Autodesk Fusion 360 part; units mm, degrees
(part 2 of 7)
sketch "Cover bearing-pad clearance sketch (3)" plane through (0, 0, 39.1) normal (0, 0, 1) x (1, 0, 0) in component "01 Shape A housing"
  circle A0 centre (77, 172) radius 4.9
  dimension "d450" = 77
  dimension "d451" = 172
  dimension "d452" = 4.9
  measures "d450" horizontal distance of origin A0.centre
  measures "d451" vertical distance of origin A0.centre
  measures "d452" radius of A0
ref_plane "WorkPlane1" through (0, 0, -8) normal (0, 0, 1) x (1, 0, 0) in component "M3 x 8 button screw — GEN-M3-BHCS-L8-AF2"
sketch "Joined screw sketch" plane through (0, 0, -8) normal (0, 0, 1) x (1, 0, 0) in component "M3 x 8 button screw — GEN-M3-BHCS-L8-AF2"
  circle A0 centre (0, 0) radius 1.45
  dimension "d457" = 1.45
  measures "d457" radius of A0
extrude "Joined screw" add sketch "Joined screw sketch" along normal blind 8 separate body makes body 17 in component "M3 x 8 button screw — GEN-M3-BHCS-L8-AF2"
ref_plane "WorkPlane2" through (0, 0, 0) normal (0, 0, 1) x (1, 0, 0) in component "M3 x 8 button screw — GEN-M3-BHCS-L8-AF2"
sketch "Screw head sketch" plane through (0, 0, 0) normal (0, 0, 1) x (1, 0, 0) in component "M3 x 8 button screw — GEN-M3-BHCS-L8-AF2"
  circle A0 centre (0, 0) radius 2.85
  dimension "d462" = 2.85
  measures "d462" radius of A0
extrude "Screw head" add sketch "Screw head sketch" along normal blind 1.65 bodies 17 in component "M3 x 8 button screw — GEN-M3-BHCS-L8-AF2"
fillet "Rounded head crown" radius 0.95 1 edges at (-2.6571, -1.0306, 1.65) on bodies 17 in component "M3 x 8 button screw — GEN-M3-BHCS-L8-AF2"
ref_plane "WorkPlane3" through (0, 0, 0.65) normal (0, 0, 1) x (1, 0, 0) in component "M3 x 8 button screw — GEN-M3-BHCS-L8-AF2"
sketch "Hex drive 2 mm across flats" plane through (0, 0, 0.65) normal (0, 0, 1) x (1, 0, 0) in component "M3 x 8 button screw — GEN-M3-BHCS-L8-AF2"
  line L0 (1.1547, 0) -> (0.5774, 1)
  line L1 (0.5774, 1) -> (-0.5774, 1)
  line L2 (-0.5774, 1) -> (-1.1547, 0)
  line L3 (-1.1547, 0) -> (-0.5774, -1)
  line L4 (-0.5774, -1) -> (0.5774, -1)
  line L5 (0.5774, -1) -> (1.1547, 0)
extrude "Hex drive recess" cut sketch "Hex drive 2 mm across flats" along normal blind 1.1 bodies 17 in component "M3 x 8 button screw — GEN-M3-BHCS-L8-AF2"
ref_plane "WorkPlane1" through (0, 0, -5) normal (0, 0, 1) x (1, 0, 0) in component "M3 insert OD4.2 x5 — GEN-M3-HEATSET-OD4.2-L5"
sketch "Hollow insert sketch" plane through (0, 0, -5) normal (0, 0, 1) x (1, 0, 0) in component "M3 insert OD4.2 x5 — GEN-M3-HEATSET-OD4.2-L5"
  circle A0 centre (0, 0) radius 2.1
  dimension "d473" = 2.1
  measures "d473" radius of A0
extrude "Hollow insert" add sketch "Hollow insert sketch" along normal blind 5 separate body makes body 18 in component "M3 insert OD4.2 x5 — GEN-M3-HEATSET-OD4.2-L5"
ref_plane "WorkPlane2" through (0, 0, -5.1) normal (0, 0, 1) x (1, 0, 0) in component "M3 insert OD4.2 x5 — GEN-M3-HEATSET-OD4.2-L5"
sketch "Unthreaded insert bore sketch" plane through (0, 0, -5.1) normal (0, 0, 1) x (1, 0, 0) in component "M3 insert OD4.2 x5 — GEN-M3-HEATSET-OD4.2-L5"
  circle A0 centre (0, 0) radius 1.55
  dimension "d478" = 1.55
  measures "d478" radius of A0
extrude "Unthreaded insert bore" cut sketch "Unthreaded insert bore sketch" along normal blind 5.2 bodies 18 in component "M3 insert OD4.2 x5 — GEN-M3-HEATSET-OD4.2-L5"
ref_plane "WorkPlane3" through (0, 0, -3.75) normal (0, 0, 1) x (1, 0, 0) in component "M3 insert OD4.2 x5 — GEN-M3-HEATSET-OD4.2-L5"
sketch "Cosmetic insert relief" plane through (0, 0, -3.75) normal (0, 0, 1) x (1, 0, 0) in component "M3 insert OD4.2 x5 — GEN-M3-HEATSET-OD4.2-L5"
  circle A0 centre (0, 0) radius 2.2
  circle A1 centre (0, 0) radius 2
  dimension "d483" = 2.2
  dimension "d484" = 2
  measures "d483" radius of A0
  measures "d484" radius of A1
extrude "Cosmetic annular relief" cut sketch "Cosmetic insert relief" along normal blind 0.25 bodies 18 in component "M3 insert OD4.2 x5 — GEN-M3-HEATSET-OD4.2-L5"
ref_plane "WorkPlane4" through (0, 0, -1.25) normal (0, 0, 1) x (1, 0, 0) in component "M3 insert OD4.2 x5 — GEN-M3-HEATSET-OD4.2-L5"
sketch "Cosmetic insert relief (1)" plane through (0, 0, -1.25) normal (0, 0, 1) x (1, 0, 0) in component "M3 insert OD4.2 x5 — GEN-M3-HEATSET-OD4.2-L5"
  circle A0 centre (0, 0) radius 2.2
  circle A1 centre (0, 0) radius 2
  dimension "d489" = 2.2
  dimension "d490" = 2
  measures "d489" radius of A0
  measures "d490" radius of A1
extrude "Cosmetic annular relief (1)" cut sketch "Cosmetic insert relief (1)" along normal blind 0.25 bodies 18 in component "M3 insert OD4.2 x5 — GEN-M3-HEATSET-OD4.2-L5"
ref_plane "WorkPlane14" through (0, 0, 38.6) normal (0, 0, 1) x (1, 0, 0) in component "02 Single rear cover"
sketch "Rear cover locating lip sketch" plane through (0, 0, 38.6) normal (0, 0, 1) x (1, 0, 0) in component "02 Single rear cover"
  line L0 (2.65, 55) -> (4.65, 55)
  line L1 (4.65, 55) -> (4.65, 67)
  line L2 (4.65, 67) -> (2.65, 67)
  line L3 (2.65, 67) -> (2.65, 55)
  dimension "d495" = 2.65
  dimension "d496" = 55
  dimension "d497" = 2
  dimension "d498" = 12
  constraint horizontal L0
  constraint vertical L1
  constraint horizontal L2
  constraint vertical L3
  measures "d495" horizontal distance of origin L0.start
  measures "d496" vertical distance of origin L0.start
  measures "d497" horizontal distance of L0.start L0.end
  measures "d498" vertical distance of L0.end L1.end
extrude "Rear cover locating lip" add sketch "Rear cover locating lip sketch" along normal blind 2.3 bodies 4 in component "02 Single rear cover"
ref_plane "WorkPlane15" through (0, 0, 38.6) normal (0, 0, 1) x (1, 0, 0) in component "02 Single rear cover"
sketch "Rear cover locating lip sketch (1)" plane through (0, 0, 38.6) normal (0, 0, 1) x (1, 0, 0) in component "02 Single rear cover"
  line L0 (2.65, 98) -> (4.65, 98)
  line L1 (4.65, 98) -> (4.65, 110)
  line L2 (4.65, 110) -> (2.65, 110)
  line L3 (2.65, 110) -> (2.65, 98)
  dimension "d503" = 2.65
  dimension "d504" = 98
  dimension "d505" = 2
  dimension "d506" = 12
  constraint horizontal L0
  constraint vertical L1
  constraint horizontal L2
  constraint vertical L3
  measures "d503" horizontal distance of origin L0.start
  measures "d504" vertical distance of origin L0.start
  measures "d505" horizontal distance of L0.start L0.end
  measures "d506" vertical distance of L0.end L1.end
extrude "Rear cover locating lip (1)" add sketch "Rear cover locating lip sketch (1)" along normal blind 2.3 bodies 4 in component "02 Single rear cover"
ref_plane "WorkPlane16" through (0, 0, 38.6) normal (0, 0, 1) x (1, 0, 0) in component "02 Single rear cover"
sketch "Rear cover locating lip sketch (2)" plane through (0, 0, 38.6) normal (0, 0, 1) x (1, 0, 0) in component "02 Single rear cover"
  line L0 (80.35, 55) -> (82.35, 55)
  line L1 (82.35, 55) -> (82.35, 67)
  line L2 (82.35, 67) -> (80.35, 67)
  line L3 (80.35, 67) -> (80.35, 55)
  dimension "d511" = 80.35
  dimension "d512" = 55
  dimension "d513" = 2
  dimension "d514" = 12
  constraint horizontal L0
  constraint vertical L1
  constraint horizontal L2
  constraint vertical L3
  measures "d511" horizontal distance of origin L0.start
  measures "d512" vertical distance of origin L0.start
  measures "d513" horizontal distance of L0.start L0.end
  measures "d514" vertical distance of L0.end L1.end
extrude "Rear cover locating lip (2)" add sketch "Rear cover locating lip sketch (2)" along normal blind 2.3 bodies 4 in component "02 Single rear cover"
ref_plane "WorkPlane17" through (0, 0, 38.6) normal (0, 0, 1) x (1, 0, 0) in component "02 Single rear cover"
sketch "Rear cover locating lip sketch (3)" plane through (0, 0, 38.6) normal (0, 0, 1) x (1, 0, 0) in component "02 Single rear cover"
  line L0 (80.35, 98) -> (82.35, 98)
  line L1 (82.35, 98) -> (82.35, 110)
  line L2 (82.35, 110) -> (80.35, 110)
  line L3 (80.35, 110) -> (80.35, 98)
  dimension "d519" = 80.35
  dimension "d520" = 98
  dimension "d521" = 2
  dimension "d522" = 12
  constraint horizontal L0
  constraint vertical L1
  constraint horizontal L2
  constraint vertical L3
  measures "d519" horizontal distance of origin L0.start
  measures "d520" vertical distance of origin L0.start
  measures "d521" horizontal distance of L0.start L0.end
  measures "d522" vertical distance of L0.end L1.end
extrude "Rear cover locating lip (3)" add sketch "Rear cover locating lip sketch (3)" along normal blind 2.3 bodies 4 in component "02 Single rear cover"
ref_plane "WorkPlane24" through (0, 0, 14.3) normal (0, 0, 1) x (1, 0, 0) in component "01 Shape A housing"
sketch "Lower battery cradle and divider anchor sketch" plane through (0, 0, 14.3) normal (0, 0, 1) x (1, 0, 0) in component "01 Shape A housing"
  line L0 (2.3, 24.5) -> (50.2, 24.5)
  line L1 (50.2, 24.5) -> (50.2, 26.5)
  line L2 (50.2, 26.5) -> (2.3, 26.5)
  line L3 (2.3, 26.5) -> (2.3, 24.5)
  dimension "d527" = 2.3
  dimension "d528" = 24.5
  dimension "d529" = 47.9
  dimension "d530" = 2
  constraint horizontal L0
  constraint vertical L1
  constraint horizontal L2
  constraint vertical L3
  measures "d527" horizontal distance of origin L0.start
  measures "d528" vertical distance of origin L0.start
  measures "d529" horizontal distance of L0.start L0.end
  measures "d530" vertical distance of L0.end L1.end
extrude "Lower battery cradle and divider anchor" add sketch "Lower battery cradle and divider anchor sketch" along normal blind 4.2 bodies 1 in component "01 Shape A housing"
ref_plane "WorkPlane25" through (0, 0, 14.3) normal (0, 0, 1) x (1, 0, 0) in component "01 Shape A housing"
sketch "Battery to PCB guide divider sketch" plane through (0, 0, 14.3) normal (0, 0, 1) x (1, 0, 0) in component "01 Shape A housing"
  line L0 (48.2, 25) -> (50.2, 25)
  line L1 (50.2, 25) -> (50.2, 117.6)
  line L2 (50.2, 117.6) -> (48.2, 117.6)
  line L3 (48.2, 117.6) -> (48.2, 25)
  dimension "d535" = 48.2
  dimension "d536" = 25
  dimension "d537" = 2
  dimension "d538" = 92.6
  constraint horizontal L0
  constraint vertical L1
  constraint horizontal L2
  constraint vertical L3
  measures "d535" horizontal distance of origin L0.start
  measures "d536" vertical distance of origin L0.start
  measures "d537" horizontal distance of L0.start L0.end
  measures "d538" vertical distance of L0.end L1.end
extrude "Battery to PCB guide divider" add sketch "Battery to PCB guide divider sketch" along normal blind 21.7 bodies 1 in component "01 Shape A housing"
ref_plane "WorkPlane26" through (0, 0, 14.3) normal (0, 0, 1) x (1, 0, 0) in component "01 Shape A housing"
sketch "Carrier fixed support web sketch" plane through (0, 0, 14.3) normal (0, 0, 1) x (1, 0, 0) in component "01 Shape A housing"
  line L0 (72.4, 24.4) -> (82.7, 24.4)
  line L1 (82.7, 24.4) -> (82.7, 31.6)
  line L2 (82.7, 31.6) -> (72.4, 31.6)
  line L3 (72.4, 31.6) -> (72.4, 24.4)
  dimension "d543" = 72.4
  dimension "d544" = 24.4
  dimension "d545" = 10.3
  dimension "d546" = 7.2
  constraint horizontal L0
  constraint vertical L1
  constraint horizontal L2
  constraint vertical L3
  measures "d543" horizontal distance of origin L0.start
  measures "d544" vertical distance of origin L0.start
  measures "d545" horizontal distance of L0.start L0.end
  measures "d546" vertical distance of L0.end L1.end
extrude "Carrier fixed support web" add sketch "Carrier fixed support web sketch" along normal blind 4.2 bodies 1 in component "01 Shape A housing"
ref_plane "WorkPlane27" through (0, 0, 14.4) normal (0, 0, 1) x (1, 0, 0) in component "01 Shape A housing"
sketch "Carrier M2 insert pilot sketch" plane through (0, 0, 14.4) normal (0, 0, 1) x (1, 0, 0) in component "01 Shape A housing"
  circle A0 centre (76, 28) radius 1.65
  dimension "d551" = 76
  dimension "d552" = 28
  dimension "d553" = 1.65
  measures "d551" horizontal distance of origin A0.centre
  measures "d552" vertical distance of origin A0.centre
  measures "d553" radius of A0
extrude "Carrier M2 insert pilot" cut sketch "Carrier M2 insert pilot sketch" along normal blind 4.2 bodies 1 in component "01 Shape A housing"
ref_plane "WorkPlane28" through (0, 0, 14.3) normal (0, 0, 1) x (1, 0, 0) in component "01 Shape A housing"
sketch "Carrier fixed support web sketch (1)" plane through (0, 0, 14.3) normal (0, 0, 1) x (1, 0, 0) in component "01 Shape A housing"
  line L0 (48.2, 110.4) -> (58.4, 110.4)
  line L1 (58.4, 110.4) -> (58.4, 117.6)
  line L2 (58.4, 117.6) -> (48.2, 117.6)
  line L3 (48.2, 117.6) -> (48.2, 110.4)
  dimension "d558" = 48.2
  dimension "d559" = 110.4
  dimension "d560" = 10.2
  dimension "d561" = 7.2
  constraint horizontal L0
  constraint vertical L1
  constraint horizontal L2
  constraint vertical L3
  measures "d558" horizontal distance of origin L0.start
  measures "d559" vertical distance of origin L0.start
  measures "d560" horizontal distance of L0.start L0.end
  measures "d561" vertical distance of L0.end L1.end
extrude "Carrier fixed support web (1)" add sketch "Carrier fixed support web sketch (1)" along normal blind 4.2 bodies 1 in component "01 Shape A housing"
ref_plane "WorkPlane29" through (0, 0, 14.4) normal (0, 0, 1) x (1, 0, 0) in component "01 Shape A housing"
sketch "Carrier M2 insert pilot sketch (1)" plane through (0, 0, 14.4) normal (0, 0, 1) x (1, 0, 0) in component "01 Shape A housing"
  circle A0 centre (54.8, 114) radius 1.65
  dimension "d566" = 54.8
  dimension "d567" = 114
  dimension "d568" = 1.65
  measures "d566" horizontal distance of origin A0.centre
  measures "d567" vertical distance of origin A0.centre
  measures "d568" radius of A0
extrude "Carrier M2 insert pilot (1)" cut sketch "Carrier M2 insert pilot sketch (1)" along normal blind 4.2 bodies 1 in component "01 Shape A housing"
ref_plane "WorkPlane1" through (0, 0, 18.5) normal (0, 0, 1) x (1, 0, 0) in component "Carrier / removable electronics tray"
sketch "PCB carrier plate sketch" plane through (0, 0, 18.5) normal (0, 0, 1) x (1, 0, 0) in component "Carrier / removable electronics tray"
  line L0 (50.2, 20.5) -> (80.6, 20.5)
  line L1 (80.6, 20.5) -> (80.6, 120.5)
  line L2 (80.6, 120.5) -> (50.2, 120.5)
  line L3 (50.2, 120.5) -> (50.2, 20.5)
  dimension "d573" = 50.2
  dimension "d574" = 20.5
  dimension "d575" = 30.4
  dimension "d576" = 100
  constraint horizontal L0
  constraint vertical L1
  constraint horizontal L2
  constraint vertical L3
  measures "d573" horizontal distance of origin L0.start
  measures "d574" vertical distance of origin L0.start
  measures "d575" horizontal distance of L0.start L0.end
  measures "d576" vertical distance of L0.end L1.end
extrude "PCB carrier plate" add sketch "PCB carrier plate sketch" along normal blind 2 separate body makes body 19 in component "Carrier / removable electronics tray"
ref_plane "WorkPlane1" through (0, 0, 20.5) normal (0, 0, 1) x (1, 0, 0) in component "Carrier / future PCB allocation — layout pending"
sketch "Future shaped PCB sketch" plane through (0, 0, 20.5) normal (0, 0, 1) x (1, 0, 0) in component "Carrier / future PCB allocation — layout pending"
  line L0 (50.4, 21) -> (80.4, 21)
  line L1 (80.4, 21) -> (80.4, 120)
  line L2 (80.4, 120) -> (50.4, 120)
  line L3 (50.4, 120) -> (50.4, 21)
  dimension "d581" = 50.4
  dimension "d582" = 21
  dimension "d583" = 30
  dimension "d584" = 99
  constraint horizontal L0
  constraint vertical L1
  constraint horizontal L2
  constraint vertical L3
  measures "d581" horizontal distance of origin L0.start
  measures "d582" vertical distance of origin L0.start
  measures "d583" horizontal distance of L0.start L0.end
  measures "d584" vertical distance of L0.end L1.end
extrude "Future shaped PCB" add sketch "Future shaped PCB sketch" along normal blind 1.6 separate body makes body 20 in component "Carrier / future PCB allocation — layout pending"
ref_plane "WorkPlane2" through (0, 0, 18.4) normal (0, 0, 1) x (1, 0, 0) in component "Carrier / removable electronics tray"
sketch "Button terminal and finger access notch sketch" plane through (0, 0, 18.4) normal (0, 0, 1) x (1, 0, 0) in component "Carrier / removable electronics tray"
  line L0 (59, 103) -> (89, 103)
  line L1 (89, 103) -> (89, 121)
  line L2 (89, 121) -> (59, 121)
  line L3 (59, 121) -> (59, 103)
  dimension "d589" = 59
  dimension "d590" = 103
  dimension "d591" = 30
  dimension "d592" = 18
  constraint horizontal L0
  constraint vertical L1
  constraint horizontal L2
  constraint vertical L3
  measures "d589" horizontal distance of origin L0.start
  measures "d590" vertical distance of origin L0.start
  measures "d591" horizontal distance of L0.start L0.end
  measures "d592" vertical distance of L0.end L1.end
extrude "Button terminal and finger access notch" cut sketch "Button terminal and finger access notch sketch" along normal blind 4 bodies 19 in component "Carrier / removable electronics tray"
ref_plane "WorkPlane3" through (0, 0, 18.4) normal (0, 0, 1) x (1, 0, 0) in component "Carrier / removable electronics tray"
sketch "Shared carrier M2 hole sketch" plane through (0, 0, 18.4) normal (0, 0, 1) x (1, 0, 0) in component "Carrier / removable electronics tray"
  circle A0 centre (76, 28) radius 1.15
  dimension "d597" = 76
  dimension "d598" = 28
  dimension "d599" = 1.15
  measures "d597" horizontal distance of origin A0.centre
  measures "d598" vertical distance of origin A0.centre
  measures "d599" radius of A0
extrude "Shared carrier M2 hole" cut sketch "Shared carrier M2 hole sketch" along normal blind 4 bodies 19 in component "Carrier / removable electronics tray"
ref_plane "WorkPlane4" through (0, 0, 18.4) normal (0, 0, 1) x (1, 0, 0) in component "Carrier / removable electronics tray"
sketch "Shared carrier M2 hole sketch (1)" plane through (0, 0, 18.4) normal (0, 0, 1) x (1, 0, 0) in component "Carrier / removable electronics tray"
  circle A0 centre (54.8, 114) radius 1.15
  dimension "d604" = 54.8
  dimension "d605" = 114
  dimension "d606" = 1.15
  measures "d604" horizontal distance of origin A0.centre
  measures "d605" vertical distance of origin A0.centre
  measures "d606" radius of A0
extrude "Shared carrier M2 hole (1)" cut sketch "Shared carrier M2 hole sketch (1)" along normal blind 4 bodies 19 in component "Carrier / removable electronics tray"
ref_plane "WorkPlane2" through (0, 0, 18.4) normal (0, 0, 1) x (1, 0, 0) in component "Carrier / future PCB allocation — layout pending"
sketch "Button terminal and finger access notch sketch (2)" plane through (0, 0, 18.4) normal (0, 0, 1) x (1, 0, 0) in component "Carrier / future PCB allocation — layout pending"
  line L0 (59, 103) -> (89, 103)
  line L1 (89, 103) -> (89, 121)
  line L2 (89, 121) -> (59, 121)
  line L3 (59, 121) -> (59, 103)
  dimension "d611" = 59
  dimension "d612" = 103
  dimension "d613" = 30
  dimension "d614" = 18
  constraint horizontal L0
  constraint vertical L1
  constraint horizontal L2
  constraint vertical L3
  measures "d611" horizontal distance of origin L0.start
  measures "d612" vertical distance of origin L0.start
  measures "d613" horizontal distance of L0.start L0.end
  measures "d614" vertical distance of L0.end L1.end
extrude "Button terminal and finger access notch'" cut sketch "Button terminal and finger access notch sketch (2)" along normal blind 4 bodies 20 in component "Carrier / future PCB allocation — layout pending"
ref_plane "WorkPlane3" through (0, 0, 18.4) normal (0, 0, 1) x (1, 0, 0) in component "Carrier / future PCB allocation — layout pending"
sketch "Shared carrier M2 hole sketch (2)" plane through (0, 0, 18.4) normal (0, 0, 1) x (1, 0, 0) in component "Carrier / future PCB allocation — layout pending"
  circle A0 centre (76, 28) radius 1.15
  dimension "d619" = 76
  dimension "d620" = 28
  dimension "d621" = 1.15
  measures "d619" horizontal distance of origin A0.centre
  measures "d620" vertical distance of origin A0.centre
  measures "d621" radius of A0
extrude "Shared carrier M2 hole'" cut sketch "Shared carrier M2 hole sketch (2)" along normal blind 4 bodies 20 in component "Carrier / future PCB allocation — layout pending"
ref_plane "WorkPlane4" through (0, 0, 18.4) normal (0, 0, 1) x (1, 0, 0) in component "Carrier / future PCB allocation — layout pending"
sketch "Shared carrier M2 hole sketch (1) (2)" plane through (0, 0, 18.4) normal (0, 0, 1) x (1, 0, 0) in component "Carrier / future PCB allocation — layout pending"
  circle A0 centre (54.8, 114) radius 1.15
  dimension "d626" = 54.8
  dimension "d627" = 114
  dimension "d628" = 1.15
  measures "d626" horizontal distance of origin A0.centre
  measures "d627" vertical distance of origin A0.centre
  measures "d628" radius of A0
extrude "Shared carrier M2 hole (1)'" cut sketch "Shared carrier M2 hole sketch (1) (2)" along normal blind 4 bodies 20 in component "Carrier / future PCB allocation — layout pending"
ref_plane "WorkPlane5" through (0, 0, 22.1) normal (0, 0, 1) x (1, 0, 0) in component "Carrier / future PCB allocation — layout pending"
sketch "Charger power zone sketch" plane through (0, 0, 22.1) normal (0, 0, 1) x (1, 0, 0) in component "Carrier / future PCB allocation — layout pending"
  line L0 (54, 37) -> (74, 37)
  line L1 (74, 37) -> (74, 60)
  line L2 (74, 60) -> (54, 60)
  line L3 (54, 60) -> (54, 37)
  dimension "d633" = 54
  dimension "d634" = 37
  dimension "d635" = 20
  dimension "d636" = 23
  constraint horizontal L0
  constraint vertical L1
  constraint horizontal L2
  constraint vertical L3
  measures "d633" horizontal distance of origin L0.start
  measures "d634" vertical distance of origin L0.start
  measures "d635" horizontal distance of L0.start L0.end
  measures "d636" vertical distance of L0.end L1.end
extrude "Charger power zone" add sketch "Charger power zone sketch" along normal blind 5 separate body makes body 21 in component "Carrier / future PCB allocation — layout pending"
ref_plane "WorkPlane6" through (0, 0, 22.1) normal (0, 0, 1) x (1, 0, 0) in component "Carrier / future PCB allocation — layout pending"
sketch "Sensor analog zone sketch" plane through (0, 0, 22.1) normal (0, 0, 1) x (1, 0, 0) in component "Carrier / future PCB allocation — layout pending"
  line L0 (54, 68) -> (74, 68)
  line L1 (74, 68) -> (74, 88)
  line L2 (74, 88) -> (54, 88)
  line L3 (54, 88) -> (54, 68)
  dimension "d641" = 54
  dimension "d642" = 68
  dimension "d643" = 20
  dimension "d644" = 20
  constraint horizontal L0
  constraint vertical L1
  constraint horizontal L2
  constraint vertical L3
  measures "d641" horizontal distance of origin L0.start
  measures "d642" vertical distance of origin L0.start
  measures "d643" horizontal distance of L0.start L0.end
  measures "d644" vertical distance of L0.end L1.end
extrude "Sensor analog zone" add sketch "Sensor analog zone sketch" along normal blind 4 separate body makes body 22 in component "Carrier / future PCB allocation — layout pending"
ref_plane "WorkPlane7" through (0, 0, 22.1) normal (0, 0, 1) x (1, 0, 0) in component "Carrier / future PCB allocation — layout pending"
sketch "Digital interface zone sketch" plane through (0, 0, 22.1) normal (0, 0, 1) x (1, 0, 0) in component "Carrier / future PCB allocation — layout pending"
  line L0 (54, 94) -> (72, 94)
  line L1 (72, 94) -> (72, 102)
  line L2 (72, 102) -> (54, 102)
  line L3 (54, 102) -> (54, 94)
  dimension "d649" = 54
  dimension "d650" = 94
  dimension "d651" = 18
  dimension "d652" = 8
  constraint horizontal L0
  constraint vertical L1
  constraint horizontal L2
  constraint vertical L3
  measures "d649" horizontal distance of origin L0.start
  measures "d650" vertical distance of origin L0.start
  measures "d651" horizontal distance of L0.start L0.end
  measures "d652" vertical distance of L0.end L1.end
extrude "Digital interface zone" add sketch "Digital interface zone sketch" along normal blind 3 separate body makes body 23 in component "Carrier / future PCB allocation — layout pending"
ref_plane "WorkPlane1" through (0, 0, -7) normal (0, 0, 1) x (1, 0, 0) in component "M2 x 7 socket_cap screw — GEN-M2-SHCS-L7-AF1.5"
sketch "Joined screw sketch (2)" plane through (0, 0, -7) normal (0, 0, 1) x (1, 0, 0) in component "M2 x 7 socket_cap screw — GEN-M2-SHCS-L7-AF1.5"
  circle A0 centre (0, 0) radius 0.95
  dimension "d657" = 0.95
  measures "d657" radius of A0
extrude "Joined screw'" add sketch "Joined screw sketch (2)" along normal blind 7 separate body makes body 24 in component "M2 x 7 socket_cap screw — GEN-M2-SHCS-L7-AF1.5"
ref_plane "WorkPlane2" through (0, 0, 0) normal (0, 0, 1) x (1, 0, 0) in component "M2 x 7 socket_cap screw — GEN-M2-SHCS-L7-AF1.5"
sketch "Screw head sketch (2)" plane through (0, 0, 0) normal (0, 0, 1) x (1, 0, 0) in component "M2 x 7 socket_cap screw — GEN-M2-SHCS-L7-AF1.5"
  circle A0 centre (0, 0) radius 1.9
  dimension "d662" = 1.9
  measures "d662" radius of A0
extrude "Screw head'" add sketch "Screw head sketch (2)" along normal blind 2 bodies 24 in component "M2 x 7 socket_cap screw — GEN-M2-SHCS-L7-AF1.5"
fillet "Rounded head crown'" radius 0.15 1 edges at (-1.7714, -0.6871, 2) on bodies 24 in component "M2 x 7 socket_cap screw — GEN-M2-SHCS-L7-AF1.5"
ref_plane "WorkPlane3" through (0, 0, 1) normal (0, 0, 1) x (1, 0, 0) in component "M2 x 7 socket_cap screw — GEN-M2-SHCS-L7-AF1.5"
sketch "Hex drive 1.5 mm across flats" plane through (0, 0, 1) normal (0, 0, 1) x (1, 0, 0) in component "M2 x 7 socket_cap screw — GEN-M2-SHCS-L7-AF1.5"
  line L0 (0.866, 0) -> (0.433, 0.75)
  line L1 (0.433, 0.75) -> (-0.433, 0.75)
  line L2 (-0.433, 0.75) -> (-0.866, 0)
  line L3 (-0.866, 0) -> (-0.433, -0.75)
  line L4 (-0.433, -0.75) -> (0.433, -0.75)
  line L5 (0.433, -0.75) -> (0.866, 0)
extrude "Hex drive recess'" cut sketch "Hex drive 1.5 mm across flats" along normal blind 1.1 bodies 24 in component "M2 x 7 socket_cap screw — GEN-M2-SHCS-L7-AF1.5"
ref_plane "WorkPlane1" through (0, 0, -4) normal (0, 0, 1) x (1, 0, 0) in component "M2 insert OD3.2 x4 — GEN-M2-HEATSET-OD3.2-L4"
sketch "Hollow insert sketch (2)" plane through (0, 0, -4) normal (0, 0, 1) x (1, 0, 0) in component "M2 insert OD3.2 x4 — GEN-M2-HEATSET-OD3.2-L4"
  circle A0 centre (0, 0) radius 1.6
  dimension "d673" = 1.6
  measures "d673" radius of A0
extrude "Hollow insert'" add sketch "Hollow insert sketch (2)" along normal blind 4 separate body makes body 25 in component "M2 insert OD3.2 x4 — GEN-M2-HEATSET-OD3.2-L4"
ref_plane "WorkPlane2" through (0, 0, -4.1) normal (0, 0, 1) x (1, 0, 0) in component "M2 insert OD3.2 x4 — GEN-M2-HEATSET-OD3.2-L4"
sketch "Unthreaded insert bore sketch (2)" plane through (0, 0, -4.1) normal (0, 0, 1) x (1, 0, 0) in component "M2 insert OD3.2 x4 — GEN-M2-HEATSET-OD3.2-L4"
  circle A0 centre (0, 0) radius 1.05
  dimension "d678" = 1.05
  measures "d678" radius of A0
extrude "Unthreaded insert bore'" cut sketch "Unthreaded insert bore sketch (2)" along normal blind 4.2 bodies 25 in component "M2 insert OD3.2 x4 — GEN-M2-HEATSET-OD3.2-L4"
ref_plane "WorkPlane3" through (0, 0, -3) normal (0, 0, 1) x (1, 0, 0) in component "M2 insert OD3.2 x4 — GEN-M2-HEATSET-OD3.2-L4"
sketch "Cosmetic insert relief (2)" plane through (0, 0, -3) normal (0, 0, 1) x (1, 0, 0) in component "M2 insert OD3.2 x4 — GEN-M2-HEATSET-OD3.2-L4"
  circle A0 centre (0, 0) radius 1.7
  circle A1 centre (0, 0) radius 1.5
  dimension "d683" = 1.7
  dimension "d684" = 1.5
  measures "d683" radius of A0
  measures "d684" radius of A1
extrude "Cosmetic annular relief'" cut sketch "Cosmetic insert relief (2)" along normal blind 0.25 bodies 25 in component "M2 insert OD3.2 x4 — GEN-M2-HEATSET-OD3.2-L4"
ref_plane "WorkPlane4" through (0, 0, -1) normal (0, 0, 1) x (1, 0, 0) in component "M2 insert OD3.2 x4 — GEN-M2-HEATSET-OD3.2-L4"
sketch "Cosmetic insert relief (1) (2)" plane through (0, 0, -1) normal (0, 0, 1) x (1, 0, 0) in component "M2 insert OD3.2 x4 — GEN-M2-HEATSET-OD3.2-L4"
  circle A0 centre (0, 0) radius 1.7
  circle A1 centre (0, 0) radius 1.5
  dimension "d689" = 1.7
  dimension "d690" = 1.5
  measures "d689" radius of A0
  measures "d690" radius of A1
extrude "Cosmetic annular relief (1)'" cut sketch "Cosmetic insert relief (1) (2)" along normal blind 0.25 bodies 25 in component "M2 insert OD3.2 x4 — GEN-M2-HEATSET-OD3.2-L4"
ref_plane "WorkPlane30" through (0, 0, 14.3) normal (0, 0, 1) x (1, 0, 0) in component "01 Shape A housing"
sketch "Lower display retainer side-wall bracket sketch" plane through (0, 0, 14.3) normal (0, 0, 1) x (1, 0, 0) in component "01 Shape A housing"
  line L0 (67.3, 8.5) -> (82.7, 8.5)
  line L1 (82.7, 8.5) -> (82.7, 16)
  line L2 (82.7, 16) -> (67.3, 16)
  line L3 (67.3, 16) -> (67.3, 8.5)
  dimension "d695" = 67.3
  dimension "d696" = 8.5
  dimension "d697" = 15.4
  dimension "d698" = 7.5
  constraint horizontal L0
  constraint vertical L1
  constraint horizontal L2
  constraint vertical L3
  measures "d695" horizontal distance of origin L0.start
  measures "d696" vertical distance of origin L0.start
  measures "d697" horizontal distance of L0.start L0.end
  measures "d698" vertical distance of L0.end L1.end
extrude "Lower display retainer side-wall bracket" add sketch "Lower display retainer side-wall bracket sketch" along normal blind 4.2 bodies 1 in component "01 Shape A housing"
ref_plane "WorkPlane31" through (0, 0, 14.3) normal (0, 0, 1) x (1, 0, 0) in component "01 Shape A housing"
sketch "Display retainer support sketch" plane through (0, 0, 14.3) normal (0, 0, 1) x (1, 0, 0) in component "01 Shape A housing"
  circle A0 centre (69, 12.3) radius 3.7
  dimension "d703" = 69
  dimension "d704" = 12.3
  dimension "d705" = 3.7
  measures "d703" horizontal distance of origin A0.centre
  measures "d704" vertical distance of origin A0.centre
  measures "d705" radius of A0
extrude "Display retainer support" add sketch "Display retainer support sketch" along normal blind 4.2 bodies 1 in component "01 Shape A housing"
ref_plane "WorkPlane32" through (0, 0, 14.4) normal (0, 0, 1) x (1, 0, 0) in component "01 Shape A housing"
sketch "Display retainer insert pilot sketch" plane through (0, 0, 14.4) normal (0, 0, 1) x (1, 0, 0) in component "01 Shape A housing"
  circle A0 centre (69, 12.3) radius 1.65
  dimension "d710" = 69
  dimension "d711" = 12.3
  dimension "d712" = 1.65
  measures "d710" horizontal distance of origin A0.centre
  measures "d711" vertical distance of origin A0.centre
  measures "d712" radius of A0
extrude "Display retainer insert pilot" cut sketch "Display retainer insert pilot sketch" along normal blind 4.2 bodies 1 in component "01 Shape A housing"
ref_plane "WorkPlane33" through (0, 0, 14.3) normal (0, 0, 1) x (1, 0, 0) in component "01 Shape A housing"
sketch "Display retainer support sketch (1)" plane through (0, 0, 14.3) normal (0, 0, 1) x (1, 0, 0) in component "01 Shape A housing"
  circle A0 centre (10.5, 126) radius 3.7
  dimension "d717" = 10.5
  dimension "d718" = 126
  dimension "d719" = 3.7
  measures "d717" horizontal distance of origin A0.centre
  measures "d718" vertical distance of origin A0.centre
  measures "d719" radius of A0
extrude "Display retainer support (1)" add sketch "Display retainer support sketch (1)" along normal blind 4.2 bodies 1 in component "01 Shape A housing"
ref_plane "WorkPlane34" through (0, 0, 14.4) normal (0, 0, 1) x (1, 0, 0) in component "01 Shape A housing"
sketch "Display retainer insert pilot sketch (1)" plane through (0, 0, 14.4) normal (0, 0, 1) x (1, 0, 0) in component "01 Shape A housing"
  circle A0 centre (10.5, 126) radius 1.65
  dimension "d724" = 10.5
  dimension "d725" = 126
  dimension "d726" = 1.65
  measures "d724" horizontal distance of origin A0.centre
  measures "d725" vertical distance of origin A0.centre
  measures "d726" radius of A0
extrude "Display retainer insert pilot (1)" cut sketch "Display retainer insert pilot sketch (1)" along normal blind 4.2 bodies 1 in component "01 Shape A housing"
ref_plane "WorkPlane1" through (0, 0, 18.5) normal (0, 0, 1) x (1, 0, 0) in component "Display / lower rear-release retainer"
sketch "Removable display retainer plate sketch" plane through (0, 0, 18.5) normal (0, 0, 1) x (1, 0, 0) in component "Display / lower rear-release retainer"
  line L0 (65.5, 7.4) -> (72.5, 7.4)
  line L1 (72.5, 7.4) -> (72.5, 16)
  line L2 (72.5, 16) -> (65.5, 16)
  line L3 (65.5, 16) -> (65.5, 7.4)
  dimension "d731" = 65.5
  dimension "d732" = 7.4
  dimension "d733" = 7
  dimension "d734" = 8.6
  constraint horizontal L0
  constraint vertical L1
  constraint horizontal L2
  constraint vertical L3
  measures "d731" horizontal distance of origin L0.start
  measures "d732" vertical distance of origin L0.start
  measures "d733" horizontal distance of L0.start L0.end
  measures "d734" vertical distance of L0.end L1.end
extrude "Removable display retainer plate" add sketch "Removable display retainer plate sketch" along normal blind 2 separate body makes body 26 in component "Display / lower rear-release retainer"
ref_plane "WorkPlane2" through (0, 0, 14.1) normal (0, 0, 1) x (1, 0, 0) in component "Display / lower rear-release retainer"
sketch "Frame contact provision sketch" plane through (0, 0, 14.1) normal (0, 0, 1) x (1, 0, 0) in component "Display / lower rear-release retainer"
  line L0 (66, 5.7) -> (72, 5.7)
  line L1 (72, 5.7) -> (72, 7.7)
  line L2 (72, 7.7) -> (66, 7.7)
  line L3 (66, 7.7) -> (66, 5.7)
  dimension "d739" = 66
  dimension "d740" = 5.7
  dimension "d741" = 6
  dimension "d742" = 2
  constraint horizontal L0
  constraint vertical L1
  constraint horizontal L2
  constraint vertical L3
  measures "d739" horizontal distance of origin L0.start
  measures "d740" vertical distance of origin L0.start
  measures "d741" horizontal distance of L0.start L0.end
  measures "d742" vertical distance of L0.end L1.end
extrude "Frame contact provision" add sketch "Frame contact provision sketch" along normal blind 6.4 bodies 26 in component "Display / lower rear-release retainer"
ref_plane "WorkPlane3" through (0, 0, 18.4) normal (0, 0, 1) x (1, 0, 0) in component "Display / lower rear-release retainer"
sketch "Retainer M2 clearance sketch" plane through (0, 0, 18.4) normal (0, 0, 1) x (1, 0, 0) in component "Display / lower rear-release retainer"
  circle A0 centre (69, 12.3) radius 1.15
  dimension "d747" = 69
  dimension "d748" = 12.3
  dimension "d749" = 1.15
  measures "d747" horizontal distance of origin A0.centre
  measures "d748" vertical distance of origin A0.centre
  measures "d749" radius of A0
extrude "Retainer M2 clearance" cut sketch "Retainer M2 clearance sketch" along normal blind 2.2 bodies 26 in component "Display / lower rear-release retainer"
ref_plane "WorkPlane1" through (0, 0, 18.5) normal (0, 0, 1) x (1, 0, 0) in component "Display / upper rear-release retainer"
sketch "Removable display retainer plate sketch (2)" plane through (0, 0, 18.5) normal (0, 0, 1) x (1, 0, 0) in component "Display / upper rear-release retainer"
  line L0 (7, 121.5) -> (14, 121.5)
  line L1 (14, 121.5) -> (14, 129.5)
  line L2 (14, 129.5) -> (7, 129.5)
  line L3 (7, 129.5) -> (7, 121.5)
  dimension "d754" = 7
  dimension "d755" = 121.5
  dimension "d756" = 7
  dimension "d757" = 8
  constraint horizontal L0
  constraint vertical L1
  constraint horizontal L2
  constraint vertical L3
  measures "d754" horizontal distance of origin L0.start
  measures "d755" vertical distance of origin L0.start
  measures "d756" horizontal distance of L0.start L0.end
  measures "d757" vertical distance of L0.end L1.end
extrude "Removable display retainer plate'" add sketch "Removable display retainer plate sketch (2)" along normal blind 2 separate body makes body 27 in component "Display / upper rear-release retainer"
ref_plane "WorkPlane2" through (0, 0, 14.1) normal (0, 0, 1) x (1, 0, 0) in component "Display / upper rear-release retainer"
sketch "Frame contact provision sketch (2)" plane through (0, 0, 14.1) normal (0, 0, 1) x (1, 0, 0) in component "Display / upper rear-release retainer"
  line L0 (8.5, 119.8) -> (12.5, 119.8)
  line L1 (12.5, 119.8) -> (12.5, 121.8)
  line L2 (12.5, 121.8) -> (8.5, 121.8)
  line L3 (8.5, 121.8) -> (8.5, 119.8)
  dimension "d762" = 8.5
  dimension "d763" = 119.8
  dimension "d764" = 4
  dimension "d765" = 2
  constraint horizontal L0
  constraint vertical L1
  constraint horizontal L2
  constraint vertical L3
  measures "d762" horizontal distance of origin L0.start
  measures "d763" vertical distance of origin L0.start
  measures "d764" horizontal distance of L0.start L0.end
  measures "d765" vertical distance of L0.end L1.end
extrude "Frame contact provision'" add sketch "Frame contact provision sketch (2)" along normal blind 6.4 bodies 27 in component "Display / upper rear-release retainer"
ref_plane "WorkPlane3" through (0, 0, 18.4) normal (0, 0, 1) x (1, 0, 0) in component "Display / upper rear-release retainer"
sketch "Retainer M2 clearance sketch (2)" plane through (0, 0, 18.4) normal (0, 0, 1) x (1, 0, 0) in component "Display / upper rear-release retainer"
  circle A0 centre (10.5, 126) radius 1.15
  dimension "d770" = 10.5
  dimension "d771" = 126
  dimension "d772" = 1.15
  measures "d770" horizontal distance of origin A0.centre
  measures "d771" vertical distance of origin A0.centre
  measures "d772" radius of A0
extrude "Retainer M2 clearance'" cut sketch "Retainer M2 clearance sketch (2)" along normal blind 2.2 bodies 27 in component "Display / upper rear-release retainer"
ref_plane "WorkPlane1" through (0, 0, -5) normal (0, 0, 1) x (1, 0, 0) in component "M2 x 5 socket_cap screw — GEN-M2-SHCS-L5-AF1.5"
sketch "Joined screw sketch (3)" plane through (0, 0, -5) normal (0, 0, 1) x (1, 0, 0) in component "M2 x 5 socket_cap screw — GEN-M2-SHCS-L5-AF1.5"
  circle A0 centre (0, 0) radius 0.95
  dimension "d777" = 0.95
  measures "d777" radius of A0
extrude "Joined screw''" add sketch "Joined screw sketch (3)" along normal blind 5 separate body makes body 28 in component "M2 x 5 socket_cap screw — GEN-M2-SHCS-L5-AF1.5"
ref_plane "WorkPlane2" through (0, 0, 0) normal (0, 0, 1) x (1, 0, 0) in component "M2 x 5 socket_cap screw — GEN-M2-SHCS-L5-AF1.5"
sketch "Screw head sketch (3)" plane through (0, 0, 0) normal (0, 0, 1) x (1, 0, 0) in component "M2 x 5 socket_cap screw — GEN-M2-SHCS-L5-AF1.5"
  circle A0 centre (0, 0) radius 1.9
  dimension "d782" = 1.9
  measures "d782" radius of A0
extrude "Screw head''" add sketch "Screw head sketch (3)" along normal blind 2 bodies 28 in component "M2 x 5 socket_cap screw — GEN-M2-SHCS-L5-AF1.5"
fillet "Rounded head crown''" radius 0.15 1 edges at (-1.7714, -0.6871, 2) on bodies 28 in component "M2 x 5 socket_cap screw — GEN-M2-SHCS-L5-AF1.5"
ref_plane "WorkPlane3" through (0, 0, 1) normal (0, 0, 1) x (1, 0, 0) in component "M2 x 5 socket_cap screw — GEN-M2-SHCS-L5-AF1.5"
sketch "Hex drive 1.5 mm across flats (2)" plane through (0, 0, 1) normal (0, 0, 1) x (1, 0, 0) in component "M2 x 5 socket_cap screw — GEN-M2-SHCS-L5-AF1.5"
  line L0 (0.866, 0) -> (0.433, 0.75)
  line L1 (0.433, 0.75) -> (-0.433, 0.75)
  line L2 (-0.433, 0.75) -> (-0.866, 0)
  line L3 (-0.866, 0) -> (-0.433, -0.75)
  line L4 (-0.433, -0.75) -> (0.433, -0.75)
  line L5 (0.433, -0.75) -> (0.866, 0)
extrude "Hex drive recess''" cut sketch "Hex drive 1.5 mm across flats (2)" along normal blind 1.1 bodies 28 in component "M2 x 5 socket_cap screw — GEN-M2-SHCS-L5-AF1.5"
ref_plane "WorkPlane1" through (0, 0, 16.5) normal (0, 0, 1) x (1, 0, 0) in component "Battery / FMA protected holder - owner-measured envelope"
sketch "Measured occupied holder outer frame sketch" plane through (0, 0, 16.5) normal (0, 0, 1) x (1, 0, 0) in component "Battery / FMA protected holder - owner-measured envelope"
  line L0 (5.4, 27) -> (47.4, 27)
  line L1 (47.4, 27) -> (47.4, 107.4)
  line L2 (47.4, 107.4) -> (5.4, 107.4)
  line L3 (5.4, 107.4) -> (5.4, 27)
  dimension "d793" = 5.4
  dimension "d794" = 27
  dimension "d795" = 42
  dimension "d796" = 80.4
  constraint horizontal L0
  constraint vertical L1
  constraint horizontal L2
  constraint vertical L3
  measures "d793" horizontal distance of origin L0.start
  measures "d794" vertical distance of origin L0.start
  measures "d795" horizontal distance of L0.start L0.end
  measures "d796" vertical distance of L0.end L1.end
extrude "Measured occupied holder outer frame" add sketch "Measured occupied holder outer frame sketch" along normal blind 20.35 separate body makes body 29 in component "Battery / FMA protected holder - owner-measured envelope"
fillet "Provisional holder outer corner rounds" radius 1 4 edges at (5.4, 107.4, 26.675) (47.4, 107.4, 26.675) (47.4, 27, 26.675) (5.4, 27, 26.675) on bodies 29 in component "Battery / FMA protected holder - owner-measured envelope"
ref_plane "WorkPlane2" through (0, 0, 17.6) normal (0, 0, 1) x (1, 0, 0) in component "Battery / FMA protected holder - owner-measured envelope"
sketch "Open occupied cell pocket sketch" plane through (0, 0, 17.6) normal (0, 0, 1) x (1, 0, 0) in component "Battery / FMA protected holder - owner-measured envelope"
  line L0 (6.4, 29) -> (46.4, 29)
  line L1 (46.4, 29) -> (46.4, 105.4)
  line L2 (46.4, 105.4) -> (6.4, 105.4)
  line L3 (6.4, 105.4) -> (6.4, 29)
  dimension "d803" = 6.4
  dimension "d804" = 29
  dimension "d805" = 40
  dimension "d806" = 76.4
  constraint horizontal L0
  constraint vertical L1
  constraint horizontal L2
  constraint vertical L3
  measures "d803" horizontal distance of origin L0.start
  measures "d804" vertical distance of origin L0.start
  measures "d805" horizontal distance of L0.start L0.end
  measures "d806" vertical distance of L0.end L1.end
extrude "Open occupied cell pocket" cut sketch "Open occupied cell pocket sketch" along normal blind 20.35 bodies 29 in component "Battery / FMA protected holder - owner-measured envelope"
ref_plane "WorkPlane1" through (0, 32, 0) normal (0, 1, 0) x (0, 0, 1) in component "Battery / 18650 cell A - owner-rated 3400 mAh"
sketch "Cell axial cylinder sketch" plane through (0, 32, 0) normal (0, 1, 0) x (1, 0, 0) in component "Battery / 18650 cell A - owner-rated 3400 mAh"
  circle A0 centre (16.2, -26.75) radius 9.1
  dimension "d811" = 16.2
  dimension "d812" = 26.75
  dimension "d813" = 9.1
  measures "d811" horizontal distance of origin A0.centre
  measures "d812" vertical distance of origin A0.centre
  measures "d813" radius of A0
extrude "Blue 18650 reference cylinder" add sketch "Cell axial cylinder sketch" along normal blind 69 separate body makes body 30 in component "Battery / 18650 cell A - owner-rated 3400 mAh"
ref_plane "WorkPlane1" through (0, 32, 0) normal (0, 1, 0) x (0, 0, 1) in component "Battery / 18650 cell B - owner-rated 3400 mAh"
sketch "Cell axial cylinder sketch (2)" plane through (0, 32, 0) normal (0, 1, 0) x (1, 0, 0) in component "Battery / 18650 cell B - owner-rated 3400 mAh"
  circle A0 centre (36.6, -26.75) radius 9.1
  dimension "d818" = 36.6
  dimension "d819" = 26.75
  dimension "d820" = 9.1
  measures "d818" horizontal distance of origin A0.centre
  measures "d819" vertical distance of origin A0.centre
  measures "d820" radius of A0
extrude "Blue 18650 reference cylinder'" add sketch "Cell axial cylinder sketch (2)" along normal blind 69 separate body makes body 31 in component "Battery / 18650 cell B - owner-rated 3400 mAh"
ref_plane "WorkPlane1" through (0, 0, 28) normal (0, 0, 1) x (1, 0, 0) in component "Battery / red RCY disconnect body - provisional reference"
sketch "Red battery disconnect reference body sketch" plane through (0, 0, 28) normal (0, 0, 1) x (1, 0, 0) in component "Battery / red RCY disconnect body - provisional reference"
  line L0 (23, 110) -> (35, 110)
  line L1 (35, 110) -> (35, 120)
  line L2 (35, 120) -> (23, 120)
  line L3 (23, 120) -> (23, 110)
  dimension "d825" = 23
  dimension "d826" = 110
  dimension "d827" = 12
  dimension "d828" = 10
  constraint horizontal L0
  constraint vertical L1
  constraint horizontal L2
  constraint vertical L3
  measures "d825" horizontal distance of origin L0.start
  measures "d826" vertical distance of origin L0.start
  measures "d827" horizontal distance of L0.start L0.end
  measures "d828" vertical distance of L0.end L1.end
extrude "Red battery disconnect reference body" add sketch "Red battery disconnect reference body sketch" along normal blind 4 separate body makes body 32 in component "Battery / red RCY disconnect body - provisional reference"
ref_plane "WorkPlane2" through (0, 0, 27.9) normal (0, 0, 1) x (1, 0, 0) in component "Battery / red RCY disconnect body - provisional reference"
sketch "Illustrative disconnect key groove sketch" plane through (0, 0, 27.9) normal (0, 0, 1) x (1, 0, 0) in component "Battery / red RCY disconnect body - provisional reference"
  line L0 (28.4, 109.9) -> (29.6, 109.9)
  line L1 (29.6, 109.9) -> (29.6, 120.1)
  line L2 (29.6, 120.1) -> (28.4, 120.1)
  line L3 (28.4, 120.1) -> (28.4, 109.9)
  dimension "d833" = 28.4
  dimension "d834" = 109.9
  dimension "d835" = 1.2
  dimension "d836" = 10.2
  constraint horizontal L0
  constraint vertical L1
  constraint horizontal L2
  constraint vertical L3
  measures "d833" horizontal distance of origin L0.start
  measures "d834" vertical distance of origin L0.start
  measures "d835" horizontal distance of L0.start L0.end
  measures "d836" vertical distance of L0.end L1.end
extrude "Illustrative disconnect key groove" cut sketch "Illustrative disconnect key groove sketch" along normal blind 0.7 bodies 32 in component "Battery / red RCY disconnect body - provisional reference"
ref_plane "WorkPlane1" through (0, 0, 32) normal (0, 0, 1) x (1, 0, 0) in component "Battery / red RCY disconnect mate - provisional reference"
sketch "Red battery disconnect mating reference sketch" plane through (0, 0, 32) normal (0, 0, 1) x (1, 0, 0) in component "Battery / red RCY disconnect mate - provisional reference"
  line L0 (23, 110) -> (35, 110)
  line L1 (35, 110) -> (35, 120)
  line L2 (35, 120) -> (23, 120)
  line L3 (23, 120) -> (23, 110)
  dimension "d841" = 23
  dimension "d842" = 110
  dimension "d843" = 12
  dimension "d844" = 10
  constraint horizontal L0
  constraint vertical L1
  constraint horizontal L2
  constraint vertical L3
  measures "d841" horizontal distance of origin L0.start
  measures "d842" vertical distance of origin L0.start
  measures "d843" horizontal distance of L0.start L0.end
  measures "d844" vertical distance of L0.end L1.end
extrude "Red battery disconnect mating reference" add sketch "Red battery disconnect mating reference sketch" along normal blind 2.2 separate body makes body 33 in component "Battery / red RCY disconnect mate - provisional reference"
ref_plane "WorkPlane35" through (0, 0, 14.3) normal (0, 0, 1) x (1, 0, 0) in component "01 Shape A housing"
sketch "Holder right guide rail sketch" plane through (0, 0, 14.3) normal (0, 0, 1) x (1, 0, 0) in component "01 Shape A housing"
  line L0 (2.3, 27) -> (4.9, 27)
  line L1 (4.9, 27) -> (4.9, 107.4)
  line L2 (4.9, 107.4) -> (2.3, 107.4)
  line L3 (2.3, 107.4) -> (2.3, 27)
  dimension "d849" = 2.3
  dimension "d850" = 27
  dimension "d851" = 2.6
  dimension "d852" = 80.4
  constraint horizontal L0
  constraint vertical L1
  constraint horizontal L2
  constraint vertical L3
  measures "d849" horizontal distance of origin L0.start
  measures "d850" vertical distance of origin L0.start
  measures "d851" horizontal distance of L0.start L0.end
  measures "d852" vertical distance of L0.end L1.end
extrude "Holder right guide rail" add sketch "Holder right guide rail sketch" along normal blind 21.7 bodies 1 in component "01 Shape A housing"
ref_plane "WorkPlane36" through (0, 0, 14.3) normal (0, 0, 1) x (1, 0, 0) in component "01 Shape A housing"
sketch "Holder end stop sketch" plane through (0, 0, 14.3) normal (0, 0, 1) x (1, 0, 0) in component "01 Shape A housing"
  line L0 (2.3, 24.5) -> (50.2, 24.5)
  line L1 (50.2, 24.5) -> (50.2, 26.5)
  line L2 (50.2, 26.5) -> (2.3, 26.5)
  line L3 (2.3, 26.5) -> (2.3, 24.5)
  dimension "d857" = 2.3
  dimension "d858" = 24.5
  dimension "d859" = 47.9
  dimension "d860" = 2
  constraint horizontal L0
  constraint vertical L1
  constraint horizontal L2
  constraint vertical L3
  measures "d857" horizontal distance of origin L0.start
  measures "d858" vertical distance of origin L0.start
  measures "d859" horizontal distance of L0.start L0.end
  measures "d860" vertical distance of L0.end L1.end
extrude "Holder end stop" add sketch "Holder end stop sketch" along normal blind 4.2 bodies 1 in component "01 Shape A housing"
ref_plane "WorkPlane37" through (0, 0, 14.3) normal (0, 0, 1) x (1, 0, 0) in component "01 Shape A housing"
sketch "Holder end stop sketch (1)" plane through (0, 0, 14.3) normal (0, 0, 1) x (1, 0, 0) in component "01 Shape A housing"
  line L0 (2.3, 107.9) -> (50.2, 107.9)
  line L1 (50.2, 107.9) -> (50.2, 109.9)
  line L2 (50.2, 109.9) -> (2.3, 109.9)
  line L3 (2.3, 109.9) -> (2.3, 107.9)
  dimension "d865" = 2.3
  dimension "d866" = 107.9
  dimension "d867" = 47.9
  dimension "d868" = 2
  constraint horizontal L0
  constraint vertical L1
  constraint horizontal L2
  constraint vertical L3
  measures "d865" horizontal distance of origin L0.start
  measures "d866" vertical distance of origin L0.start
  measures "d867" horizontal distance of L0.start L0.end
  measures "d868" vertical distance of L0.end L1.end
extrude "Holder end stop (1)" add sketch "Holder end stop sketch (1)" along normal blind 4.2 bodies 1 in component "01 Shape A housing"
ref_plane "WorkPlane38" through (0, 0, 14.3) normal (0, 0, 1) x (1, 0, 0) in component "01 Shape A housing"